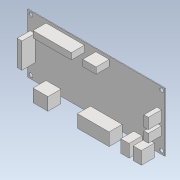
# Autodesk Inventor part: Плата контроллера
Saved by Autodesk Inventor 2021.2 (Build 252289000, 289)
## iProperties
Created: 2022-12-01
Part Number: Плата контроллера
Material: Типовые
Document SubType Name: ЛистМат
Designer: Voodoo
Mass: 17.1979 g
Surface Area: 152.475 cm^2
Volume: 17.1979 cm^3
Density: 1 g/cm^3
Sheet Metal Rule: По умолчанию_мм
Appearance: По умолчанию
Author: Voodoo
Autodesk Inventor part; units mm, degrees
ref_plane "YZ Plane" through (0, 0, 0) normal (1, 0, 0) x (0, 1, 0)
ref_plane "XZ Plane" through (0, 0, 0) normal (0, 1, 0) x (-1, 0, 0)
ref_plane "XY Plane" through (0, 0, 0) normal (0, 0, 1) x (1, 0, 0)
sketch "Эскиз1" plane through (0, 0, 0) normal (0, 0, 1) x (1, 0, 0)
  line L0 (0, 0) -> (105, 0)
  line L1 (105, 0) -> (105, 45)
  line L2 (105, 45) -> (0, 45)
  line L3 (0, 45) -> (0, 0)
  line L4 (2.5, 2.5) -> (102.5, 2.5) construction
  line L5 (102.5, 2.5) -> (102.5, 42.5) construction
  line L6 (102.5, 42.5) -> (2.5, 42.5) construction
  line L7 (2.5, 42.5) -> (2.5, 2.5) construction
  circle A0 centre (2.5, 2.5) radius 1.5
  circle A1 centre (2.5, 42.5) radius 1.5
  circle A2 centre (102.5, 42.5) radius 1.5
  circle A3 centre (102.5, 2.5) radius 1.5
  dimension "d0" = 45
  dimension "d1" = 105
  dimension "d2" = 2.5
  dimension "d3" = 3
  dimension "d4" = 3
  dimension "d5" = 3
  dimension "d6" = 3
  measures "d0" distance of L2.end L0.start
  measures "d1" distance of L0.start L0.end
  measures "d2" distance between parallel lines of L3 L7
  measures "d3" diameter of A0
  measures "d4" diameter of A1
  measures "d5" diameter of A2
  measures "d6" diameter of A3
extrude "Пластина1" add sketch "Эскиз1" along normal blind 2
sketch "Эскиз2" plane through (0, 0, 2) normal (0, 0, 1) x (1, 0, 0)
  circle A0 centre (102.5, 2.5) radius 1.5 projected
  circle A1 centre (102.5, 42.5) radius 1.5 projected
  circle A2 centre (2.5, 42.5) radius 1.5 projected
  circle A3 centre (2.5, 2.5) radius 1.5 projected
  line L0 (0, 0) -> (0, 45) projected
  line L1 (105, 0) -> (0, 0) projected
  line L2 (105, 45) -> (105, 0) projected
  line L3 (0, 45) -> (105, 45) projected
  line L4 (97.0825, -4.8574) -> (90.7781, -4.8574)
  line L5 (90.7781, -4.8574) -> (90.7781, 4.8417)
  line L6 (90.7781, 4.8417) -> (97.0825, 4.8417)
  line L7 (97.0825, 4.8417) -> (97.0825, -4.8574)
  line L8 (87.6259, -4.8574) -> (81.3215, -4.8574)
  line L9 (81.3215, -4.8574) -> (81.3215, 4.8417)
  line L10 (81.3215, 4.8417) -> (87.6259, 4.8417)
  line L11 (87.6259, 4.8417) -> (87.6259, -4.8574)
  line L12 (72.3499, -4.8574) -> (48.1023, -4.8574)
  line L13 (48.1023, -4.8574) -> (48.1023, 4.8417)
  line L14 (48.1023, 4.8417) -> (72.3499, 4.8417)
  line L15 (72.3499, 4.8417) -> (72.3499, -4.8574)
  line L16 (25.552, -4.8574) -> (14.1556, -4.8574)
  line L17 (14.1556, -4.8574) -> (14.1556, 4.8417)
  line L18 (14.1556, 4.8417) -> (25.552, 4.8417)
  line L19 (25.552, 4.8417) -> (25.552, -4.8574)
  line L20 (43.4953, 38.0609) -> (14.1556, 38.0609)
  line L21 (14.1556, 38.0609) -> (14.1556, 42.9104)
  line L22 (14.1556, 42.9104) -> (43.4953, 42.9104)
  line L23 (43.4953, 42.9104) -> (43.4953, 38.0609)
  line L24 (62.4084, 38.0609) -> (52.2244, 38.0609)
  line L25 (52.2244, 38.0609) -> (52.2244, 42.9104)
  line L26 (52.2244, 42.9104) -> (62.4084, 42.9104)
  line L27 (62.4084, 42.9104) -> (62.4084, 38.0609)
  line L28 (102.417, 12.3584) -> (99.0223, 12.3584)
  line L29 (99.0223, 12.3584) -> (99.0223, 18.9053)
  line L30 (99.0223, 18.9053) -> (102.417, 18.9053)
  line L31 (102.417, 18.9053) -> (102.417, 12.3584)
  line L32 (102.417, 21.3301) -> (99.0223, 21.3301)
  line L33 (99.0223, 21.3301) -> (99.0223, 29.5742)
  line L34 (99.0223, 29.5742) -> (102.417, 29.5742)
  line L35 (102.417, 29.5742) -> (102.417, 21.3301)
  line L36 (5.669, 12.3584) -> (2.0318, 12.3584)
  line L37 (2.0318, 12.3584) -> (2.0318, 31.7565)
  line L38 (2.0318, 31.7565) -> (5.669, 31.7565)
  line L39 (5.669, 31.7565) -> (5.669, 12.3584)
  constraints: 72 end point, 18 parallel, 12 point on line, 9 horizontal, 9 perpendicular
extrude "Выдавливание1" add sketch "Эскиз2" along normal blind 10 separate body contours L17 L18 L19 L1 | L1 L19 L16 L17 | L13 L14 L15 L1 | L1 L15 L12 L13 | L7 L4 L5 L1 | L1 L5 L6 L7 | L9 L10 L11 L1 | L1 L11 L8 L9 | L20 L21 L22 L23 | L24 L25 L26 L27 | L28 L29 L30 L31 | L32 L33 L34 L35 | L36 L37 L38 L39
equation "\"d7\" = Толщина"
equation "\"Радиус_гибки\" = Толщина"
equation "\"Ширина_просечки\" = Толщина"
equation "\"Глубина_просечки\" = 0.5 * Толщина"
equation "\"Размер_просечки\" = 4 * Толщина"
equation "\"Мин_остаток\" = 2 * Толщина"
equation "\"Радиус_перехода\" = Радиус_гибки"
equation "\"Радиус_Якоби\" = Радиус_гибки"
equation "\"Размер_зазора\" = Толщина"
equation "\"Толщина\" = 2"
